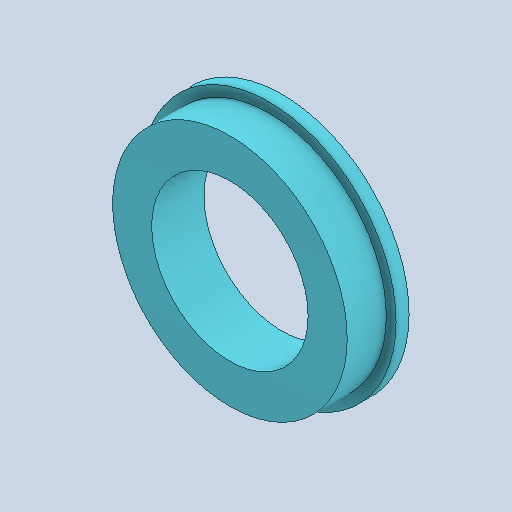
# Autodesk Inventor part: TH22_bearing_12_18_19.5_sn
Saved by Autodesk Inventor 2025.1 (Build 291241000, 241)
## iProperties
Created: 2021-10-05
Part Number: TH22_bearing_12_18_19.5_sn
Material: アルミニウム 6061-AHC
Document SubType Name: Modeling
Designer: 中島 青蔵
Density: 2.7 g/cm^3
Appearance: くすんだ青
Author: 中島 青蔵
Autodesk Inventor part; units mm, degrees
ref_plane "YZ Plane" through (0, 0, 0) normal (1, 0, 0) x (0, 1, 0)
ref_plane "XZ Plane" through (0, 0, 0) normal (0, 1, 0) x (-1, 0, 0)
ref_plane "XY Plane" through (0, 0, 0) normal (0, 0, 1) x (1, 0, 0)
sketch "スケッチ1" plane through (0, 0, 0) normal (0, 0, 1) x (1, 0, 0)
  circle A0 centre (0, 0) radius 6
  circle A1 centre (0, 0) radius 9
  circle A2 centre (0, 0) radius 9.75
  dimension "d0" = 12
  dimension "d1" = 18
  dimension "d2" = 19.5
  constraints: 3 centre point, 3 coincident
  measures "d0" diameter of A0
  measures "d1" diameter of A1
  measures "d2" diameter of A2
extrude "押し出し1" add sketch "スケッチ1" along normal blind 1 contours A2
extrude "押し出し2" add sketch "スケッチ1" along normal blind 4 contours A1
